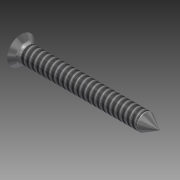
# Autodesk Inventor part: Wettterstation_Schraube
Saved by Autodesk Inventor 2014 SP1 (Build 180222100, 222)
## iProperties
Created: 2016-11-19
Part Number: Wettterstation_Schraube
Material: Edelstahl
Document SubType Name: Modeling
Designer: Flo
Density: 8.08 g/cm^3
Appearance: Halbpoliert
Author: Flo
Autodesk Inventor part; units mm, degrees
ref_plane "YZ Plane" through (0, 0, 0) normal (1, 0, 0) x (0, 1, 0)
ref_plane "XZ Plane" through (0, 0, 0) normal (0, 1, 0) x (-1, 0, 0)
ref_plane "XY Plane" through (0, 0, 0) normal (0, 0, 1) x (1, 0, 0)
sketch "Skizze1" plane through (0, 0, 0) normal (0, 1, 0) x (-1, 0, 0)
  line L0 (0, 0) -> (21.1609, 0)
  line L1 (0, 0) -> (-2.4249, 1.4)
  line L2 (0, 0) -> (2.8, 0) construction
  line L3 (21.868, -0.2929) -> (22.5751, -1)
  line L4 (-2.4249, 1.4) -> (-2.4249, 1.5)
  line L5 (-2.4249, 1.5) -> (22.5751, 1.5)
  line L6 (22.5751, -1) -> (22.5751, 1.5)
  arc A0 (21.868, -0.2929) -> (21.1609, 0) centre (21.1609, -1) ccw
  point P0 (21.5751, 0)
  dimension "d22" = 0.1
  dimension "d23" = 25
  dimension "d32" = 1
  dimension "d52" = 1.5
  dimension "d53" = 135
  dimension "d54" = 2.5
  dimension "d55" = 30
  constraints: 14 end point, 2 horizontal, 2 perpendicular, 2 point on circle, 2 point on line, 2 tangent, 1 centre point, 1 equal length, 1 parallel
  measures "d22" distance of L1.end L4.end
  measures "d23" distance of L4.end L5.end
  measures "d32" radius of A0
  measures "d52" distance between parallel lines of L5 L0
  measures "d53" angle of L3 L0
  measures "d54" distance from line of L3.end L5
  measures "d55" angle of L5 L1
revolve "Umdrehung1" add sketch "Skizze1" angle 360 about axis through (2.4249, 0, 1.5) along (-1, 0, 0)
thread "Gewinde1" size "R 1/16" standard "ISO Taper" length 21
sketch "Skizze2" plane through (-22.5751, 0, 1.5) normal (-1, 0, 0) x (0, 0, 1)
  circle A0 centre (0, 0) radius 0.0008 projected
  line L0 (0.4, 1.8) -> (-0.4, 1.8)
  line L1 (0.4, -1.8) -> (-0.4, -1.8)
  line L2 (1.8, 0.4) -> (1.8, -0.4)
  line L3 (-1.8, 0.4) -> (-1.8, -0.4)
  line L4 (-1.8, -0.4) -> (-0.4, -0.4)
  line L5 (-1.8, 0.4) -> (-0.4, 0.4)
  line L6 (1.8, 0.4) -> (0.4, 0.4)
  line L7 (1.8, -0.4) -> (0.4, -0.4)
  line L8 (0.4, -1.8) -> (0.4, -0.4)
  line L9 (0.4, 0.4) -> (0.4, 1.8)
  line L10 (-0.4, -1.8) -> (-0.4, -0.4)
  line L11 (-0.4, 0.4) -> (-0.4, 1.8)
  point P0 (-1.5, 0)
  dimension "d48" = 0.8
  dimension "d49" = 0.8
  dimension "d56" = 1.8
  dimension "d57" = 1.8
  dimension "d58" = 1.8
  dimension "d59" = 1.8
  dimension "d61" = 0.8
  dimension "d62" = 0.8
  dimension "d63" = 0.4
  dimension "d64" = 0.4
  dimension "d65" = 0.4
  dimension "d66" = 0.4
  constraints: 24 end point, 8 parallel, 8 perpendicular, 1 collinear, 1 horizontal
  measures "d48" distance of L0.start L0.end
  measures "d49" distance of L2.start L2.end
  measures "d56" distance from line of L2 A0.centre
  measures "d57" distance from line of L3 A0.centre
  measures "d58" distance from line of L1 A0.centre
  measures "d59" distance from line of L0 A0.centre
  measures "d61" distance between parallel lines of L10 L8
  measures "d62" distance between parallel lines of L5 L4
  measures "d63" distance from line of L9 A0.centre
  measures "d64" distance from line of A0.centre L4
  measures "d65" distance from line of A0.centre L10
  measures "d66" distance from line of A0.centre L7
extrude "Extrusion2" cut sketch "Skizze2" against normal blind 0.6
